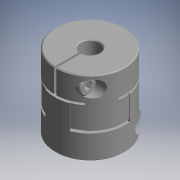
# Autodesk Inventor part: 562682 EAMC-30-32-8-14
Saved by Autodesk Inventor 2017.3 (Build 213256000, 256)
## iProperties
Part Number: 562682 EAMC-30-32-8-14
Material: Generic
Catalog Web Link: www.cadenas.de
Description: EAMC-Coupling
Vendor: FESTO
Document SubType Name: Modeling
Designer: partserver
Manufacturer: FESTO
Mass: 48 g
Surface Area: 90.1737 cm^2
Volume: 17.1118 cm^3
Density: 1 g/cm^3
Appearance: PSOLRGB-192-192-192
Category: PARTsolutions
Company: FESTO
Title: 562682 EAMC-30-32-8-14
Author: Cadenas PARTsolutions
Comments: Coupling
PSOL_IDENT_0: {$CADENAS_DATA\23d-libs\festo\parts\e\eamc\eamc.prj},183 {VTYP=3D},{NB=562682 EAMC-30-32-8-14},{LINA=
PSOL_IDENT_1: 562682 EAMC-30-32-8-14},{NN=EAMC},{DATE=08.03.2021 06:21:26},{GEOMDATE=08.03.2021 06:21:00},{VERSION=
PSOL_IDENT_2: },{LINEID=980},{WBVAR=},{WBNUMERIC=}  {NB=562682 EAMC-30-32-8-14},{LINA=562682 EAMC-30-32-8-14},{KT=
PSOL_IDENT_3: DUMMY},{TNR=562682},{TYP=EAMC-30-32-8-14},{INFO=},{CNSMASSEXACT=0.048},{VERS=7.000},{VERS2=0.000},{D=
PSOL_IDENT_4: 14},{D1=8.00},{D2=14.00},{D3=0.000},{D4=0.000},{L1=0.000},{L2=0.000},{L3=0.000},{L4=0.000},{L5=0.000
PSOL_IDENT_5: },{L6=0.000},{X=0.000},{EOLDATE=},{DI=14.200}
NB: 562682 EAMC-30-32-8-14
NN: EAMC
NT: Coupling
NBSYN: $TNR. $TYP.
LINA: 562682 EAMC-30-32-8-14
CATALOG: Festo
TNR: 562682
TYP: EAMC-30-32-8-14
CNSMASSEXACT: 0.048
D: 14
D1: 8
D2: 14
D3: 0
L1: 0
L2: 0
L3: 0
DI: 14.2
SUPPLIER: FESTO
ARTICLENO: 562682 EAMC-30-32-8-14
BOMINFO: 562682 EAMC-30-32-8-14
CREATOR: CADENAS GmbH
Autodesk Inventor part; units mm, degrees
sketch "Sketch_1" plane through (0, 0, 0) normal (1, 0, 0) x (0, 1, 0)
  line L0 (0, 10.3) -> (0, 0)
  line L1 (0, 0) -> (-15, 0)
  line L2 (-15, 0) -> (-15, 10.3)
  line L3 (-15, 10.3) -> (0, 10.3)
  line L4 (0, 10.3) -> (0, 0)
  constraints: 10 end point
revolve "Revolution1" add sketch "Sketch_1" angle 360 about axis through (0, 0, 10.3) along (0, 0, -1)
sketch "Sketch_2" plane through (0, 0, 9.3) normal (0, 0, 1) x (1, 0, 0)
  line L0 (-5.831, 14.8996) -> (-2.8531, 9.7417)
  arc A0 (-2.8531, 9.7417) -> (-0.9134, 8.7525) centre (-1.121, 10.7417) ccw
  arc A1 (0.9134, 8.7525) -> (-0.9134, 8.7525) centre (0, 0) ccw
  arc A2 (0.9134, 8.7525) -> (2.8531, 9.7417) centre (1.121, 10.7417) ccw
  line L1 (2.8531, 9.7417) -> (5.831, 14.8996)
  arc A3 (5.831, 14.8996) -> (-5.831, 14.8996) centre (0, 0) ccw
  constraints: 8 point on circle, 4 centre point, 4 end point
extrude "Extrusion1" add sketch "Sketch_2" along normal blind 11.4
sketch "Sketch_3" plane through (0, 0, 10.3) normal (0, 0, 1) x (1, 0, 0)
  arc A0 (-15.819, -2.4) -> (-9.9879, -12.4996) centre (0, 0) ccw
  line L0 (-9.9879, -12.4996) -> (-7.01, -7.3417)
  arc A1 (-7.01, -7.3417) -> (-7.1231, -5.1673) centre (-8.742, -6.3417) ccw
  arc A2 (-8.0366, -3.5852) -> (-7.1231, -5.1673) centre (0, 0) ccw
  arc A3 (-8.0366, -3.5852) -> (-9.8631, -2.4) centre (-9.8631, -4.4) ccw
  line L1 (-9.8631, -2.4) -> (-15.819, -2.4)
  constraints: 8 point on circle, 4 centre point, 4 end point
extrude "Extrusion2" add sketch "Sketch_3" along normal blind 10.4
sketch "Sketch_24" plane through (0, 0, 10.3) normal (0, 0, 1) x (1, 0, 0)
  arc A0 (7.1231, -5.1673) -> (7.01, -7.3417) centre (8.742, -6.3417) ccw
  line L0 (7.01, -7.3417) -> (9.9879, -12.4996)
  arc A1 (9.9879, -12.4996) -> (15.819, -2.4) centre (0, 0) ccw
  line L1 (15.819, -2.4) -> (9.8631, -2.4)
  arc A2 (9.8631, -2.4) -> (8.0366, -3.5852) centre (9.8631, -4.4) ccw
  arc A3 (7.1231, -5.1673) -> (8.0366, -3.5852) centre (0, 0) ccw
  constraints: 8 point on circle, 4 centre point, 4 end point
extrude "Extrusion3" add sketch "Sketch_24" along normal blind 10.4
sketch "Sketch_4" plane through (0, 0, 20.7) normal (0, 0, 1) x (1, 0, 0)
  arc A0 (-14.6202, 2.3) -> (-14.6202, -2.3) centre (0, 0) ccw
  line L0 (-14.6202, -2.3) -> (-10.016, -2.3)
  arc A1 (-8.1782, -3.511) -> (-10.016, -2.3) centre (-10.016, -4.3) ccw
  arc A2 (-8.1782, -3.511) -> (-7.1297, -5.327) centre (0, 0) ccw
  arc A3 (-6.9999, -7.5241) -> (-7.1297, -5.327) centre (-8.7319, -6.5241) ccw
  line L1 (-6.9999, -7.5241) -> (-9.302, -11.5115)
  arc A4 (-9.302, -11.5115) -> (-5.3182, -13.8115) centre (0, 0) ccw
  line L2 (-5.3182, -13.8115) -> (-3.0161, -9.8241)
  arc A5 (-1.0485, -8.838) -> (-3.0161, -9.8241) centre (-1.2841, -10.8241) ccw
  arc A6 (-1.0485, -8.838) -> (1.0485, -8.838) centre (0, 0) ccw
  arc A7 (3.0161, -9.8241) -> (1.0485, -8.838) centre (1.2841, -10.8241) ccw
  line L3 (3.0161, -9.8241) -> (5.3182, -13.8115)
  arc A8 (5.3182, -13.8115) -> (9.302, -11.5115) centre (0, 0) ccw
  line L4 (9.302, -11.5115) -> (6.9999, -7.5241)
  arc A9 (7.1297, -5.327) -> (6.9999, -7.5241) centre (8.7319, -6.5241) ccw
  arc A10 (7.1297, -5.327) -> (8.1782, -3.511) centre (0, 0) ccw
  arc A11 (10.016, -2.3) -> (8.1782, -3.511) centre (10.016, -4.3) ccw
  line L5 (10.016, -2.3) -> (14.6202, -2.3)
  arc A12 (14.6202, -2.3) -> (14.6202, 2.3) centre (0, 0) ccw
  line L6 (14.6202, 2.3) -> (10.016, 2.3)
  arc A13 (8.1782, 3.511) -> (10.016, 2.3) centre (10.016, 4.3) ccw
  arc A14 (8.1782, 3.511) -> (7.1297, 5.327) centre (0, 0) ccw
  arc A15 (6.9999, 7.5241) -> (7.1297, 5.327) centre (8.7319, 6.5241) ccw
  line L7 (6.9999, 7.5241) -> (9.302, 11.5115)
  arc A16 (9.302, 11.5115) -> (5.3182, 13.8115) centre (0, 0) ccw
  line L8 (5.3182, 13.8115) -> (3.0161, 9.8241)
  arc A17 (1.0485, 8.838) -> (3.0161, 9.8241) centre (1.2841, 10.8241) ccw
  arc A18 (1.0485, 8.838) -> (-1.0485, 8.838) centre (0, 0) ccw
  arc A19 (-3.0161, 9.8241) -> (-1.0485, 8.838) centre (-1.2841, 10.8241) ccw
  line L9 (-3.0161, 9.8241) -> (-5.3182, 13.8115)
  arc A20 (-5.3182, 13.8115) -> (-9.302, 11.5115) centre (0, 0) ccw
  line L10 (-9.302, 11.5115) -> (-6.9999, 7.5241)
  arc A21 (-7.1297, 5.327) -> (-6.9999, 7.5241) centre (-8.7319, 6.5241) ccw
  arc A22 (-7.1297, 5.327) -> (-8.1782, 3.511) centre (0, 0) ccw
  arc A23 (-10.016, 2.3) -> (-8.1782, 3.511) centre (-10.016, 4.3) ccw
  line L11 (-10.016, 2.3) -> (-14.6202, 2.3)
  constraints: 48 point on circle, 24 centre point, 24 end point
extrude "Extrusion4" add sketch "Sketch_4" against normal blind 9.4
sketch "Sketch_5" plane through (0, 0, 21.2) normal (0, 0, 1) x (1, 0, 0)
  circle A0 centre (6.132, -10.617) radius 1
  constraints: 1 centre point
extrude "Extrusion5" add sketch "Sketch_5" against normal blind 10.5
sketch "Sketch_6" plane through (0, 0, 21.2) normal (0, 0, 1) x (1, 0, 0)
  circle A0 centre (12.2606, 0.002) radius 1
  constraints: 1 centre point
extrude "Extrusion6" add sketch "Sketch_6" against normal blind 10.5
sketch "Sketch_25" plane through (0, 0, 21.2) normal (0, 0, 1) x (1, 0, 0)
  circle A0 centre (6.1286, 10.619) radius 1
  constraints: 1 centre point
extrude "Extrusion7" add sketch "Sketch_25" against normal blind 10.5
sketch "Sketch_26" plane through (0, 0, 21.2) normal (0, 0, 1) x (1, 0, 0)
  circle A0 centre (-6.132, 10.617) radius 1
  constraints: 1 centre point
extrude "Extrusion8" add sketch "Sketch_26" against normal blind 10.5
sketch "Sketch_27" plane through (0, 0, 21.2) normal (0, 0, 1) x (1, 0, 0)
  circle A0 centre (-12.2606, -0.002) radius 1
  constraints: 1 centre point
extrude "Extrusion9" add sketch "Sketch_27" against normal blind 10.5
sketch "Sketch_28" plane through (0, 0, 21.2) normal (0, 0, 1) x (1, 0, 0)
  circle A0 centre (-6.1286, -10.619) radius 1
  constraints: 1 centre point
extrude "Extrusion10" add sketch "Sketch_28" against normal blind 10.5
sketch "Sketch_7" plane through (0, 0, 11.3) normal (0, 0, 1) x (1, 0, 0)
  line L0 (-15.819, 2.4) -> (-9.8631, 2.4)
  arc A0 (-9.8631, 2.4) -> (-8.0366, 3.5852) centre (-9.8631, 4.4) ccw
  arc A1 (-7.1231, 5.1673) -> (-8.0366, 3.5852) centre (0, 0) ccw
  arc A2 (-7.1231, 5.1673) -> (-7.01, 7.3417) centre (-8.742, 6.3417) ccw
  line L1 (-7.01, 7.3417) -> (-9.9879, 12.4996)
  arc A3 (-9.9879, 12.4996) -> (-15.819, 2.4) centre (0, 0) ccw
  constraints: 8 point on circle, 4 centre point, 4 end point
extrude "Extrusion11" add sketch "Sketch_7" along normal blind 11
sketch "Sketch_8" plane through (0, 0, 11.3) normal (0, 0, 1) x (1, 0, 0)
  arc A0 (-5.831, -14.8996) -> (5.831, -14.8996) centre (0, 0) ccw
  line L0 (5.831, -14.8996) -> (2.8531, -9.7417)
  arc A1 (2.8531, -9.7417) -> (0.9134, -8.7525) centre (1.121, -10.7417) ccw
  arc A2 (-0.9134, -8.7525) -> (0.9134, -8.7525) centre (0, 0) ccw
  arc A3 (-0.9134, -8.7525) -> (-2.8531, -9.7417) centre (-1.121, -10.7417) ccw
  line L1 (-2.8531, -9.7417) -> (-5.831, -14.8996)
  constraints: 8 point on circle, 4 centre point, 4 end point
extrude "Extrusion12" add sketch "Sketch_8" along normal blind 11
sketch "Sketch_29" plane through (0, 0, 11.3) normal (0, 0, 1) x (1, 0, 0)
  arc A0 (7.01, 7.3417) -> (7.1231, 5.1673) centre (8.742, 6.3417) ccw
  arc A1 (8.0366, 3.5852) -> (7.1231, 5.1673) centre (0, 0) ccw
  arc A2 (8.0366, 3.5852) -> (9.8631, 2.4) centre (9.8631, 4.4) ccw
  line L0 (9.8631, 2.4) -> (15.819, 2.4)
  arc A3 (15.819, 2.4) -> (9.9879, 12.4996) centre (0, 0) ccw
  line L1 (9.9879, 12.4996) -> (7.01, 7.3417)
  constraints: 8 point on circle, 4 centre point, 4 end point
extrude "Extrusion13" add sketch "Sketch_29" along normal blind 11
sketch "Sketch_9" plane through (0, 0, 0) normal (1, 0, 0) x (0, 1, 0)
  line L0 (0, 32) -> (0, 21.7)
  line L1 (0, 21.7) -> (-15, 21.7)
  line L2 (-15, 21.7) -> (-15, 32)
  line L3 (-15, 32) -> (0, 32)
  line L4 (0, 32) -> (0, 21.7)
  constraints: 10 end point
revolve "Revolution2" add sketch "Sketch_9" angle 360 about axis through (0, 0, 32) along (0, 0, -1)
sketch "Sketch_10" plane through (0, 0, 0) normal (1, 0, 0) x (0, 1, 0)
  line L0 (0, 32) -> (0, 0)
  line L1 (-14.6, 32) -> (-17, 32)
  line L2 (-17, 32) -> (-17, 0)
  line L3 (-17, 0) -> (-14.6, 0)
  line L4 (-14.6, 0) -> (-15, 0.4)
  line L5 (-15, 0.4) -> (-15, 31.6)
  line L6 (-15, 31.6) -> (-14.6, 32)
  constraints: 14 end point
revolve "Revolution3" cut sketch "Sketch_10" angle 360 about axis through (0, 0, 32) along (0, 0, -1)
sketch "Sketch_11" plane through (0, 0, 0) normal (1, 0, 0) x (0, 1, 0)
  line L0 (0, 32) -> (0, 0)
  line L1 (0, 0) -> (-4.4, 0)
  line L2 (-4.4, 0) -> (-4, 0.4)
  line L3 (-4, 0.4) -> (-4, 9.8)
  line L4 (-4, 9.8) -> (-8.3, 9.8)
  arc A0 (-8.8, 10.3) -> (-8.3, 9.8) centre (-8.3, 10.3) ccw
  line L5 (-8.8, 10.3) -> (-8.8, 11.25)
  line L6 (-8.8, 11.25) -> (-7.1, 11.25)
  line L7 (-7.1, 11.25) -> (-7.1, 20.75)
  line L8 (-7.1, 20.75) -> (-8.8, 20.75)
  line L9 (-8.8, 20.75) -> (-8.8, 22.1)
  arc A1 (-8.3, 22.6) -> (-8.8, 22.1) centre (-8.3, 22.1) ccw
  line L10 (-8.3, 22.6) -> (-7, 22.6)
  line L11 (-7, 22.6) -> (-7, 31.6)
  line L12 (-7, 31.6) -> (-7.4, 32)
  line L13 (-7.4, 32) -> (0, 32)
  line L14 (0, 32) -> (0, 0)
  constraints: 30 end point, 4 point on circle, 2 centre point
revolve "Revolution4" cut sketch "Sketch_11" angle 360 about axis through (0, 0, 32) along (0, 0, -1)
sketch "Sketch_20" plane through (0, 0, 0) normal (0, 0, 1) x (1, 0, 0)
  line L0 (-0.5, -16) -> (0.5, -16)
  line L1 (0.5, -16) -> (0.5, 0)
  line L2 (0.5, 0) -> (-0.5, 0)
  line L3 (-0.5, 0) -> (-0.5, -16)
  constraints: 8 end point
extrude "Extrusion14" cut sketch "Sketch_20" along normal blind 10.3
sketch "Sketch_21" plane through (0, 0, 32) normal (0, 0, 1) x (1, 0, 0)
  line L0 (-0.5, 0) -> (0.5, 0)
  line L1 (0.5, 0) -> (0.5, 16)
  line L2 (0.5, 16) -> (-0.5, 16)
  line L3 (-0.5, 16) -> (-0.5, 0)
  constraints: 8 end point
extrude "Extrusion15" cut sketch "Sketch_21" against normal blind 10.3
sketch "Sketch_13" plane through (0, 0, 5.1) normal (0, 0, 1) x (1, 0, 0)
  line L0 (-16.5, -9.8) -> (13.5, -9.8)
  line L1 (13.5, -9.8) -> (13.5, -11.8)
  line L2 (13.5, -11.8) -> (13.121, -11.421)
  line L3 (13.121, -11.421) -> (-4.721, -11.421)
  line L4 (-4.721, -11.421) -> (-5.1, -11.8)
  line L5 (-5.1, -11.8) -> (-5.1, -13.3)
  line L6 (-5.1, -13.3) -> (-16.5, -13.3)
  line L7 (-16.5, -13.3) -> (-16.5, -9.8)
  line L8 (-16.5, -9.8) -> (13.5, -9.8)
  constraints: 18 end point
revolve "Revolution5" cut sketch "Sketch_13" angle 360 about axis through (-16.5, -9.8, 5.1) along (-1, 0, 0)
thread "Thread1" size "M4x0.7" class "6H" standard "ISO Metric profile" length 17.842
sketch "Sketch_15" plane through (0, 0, 5.1) normal (0, 0, 1) x (1, 0, 0)
  line L0 (-9.1, -9.8) -> (6.9, -9.8)
  line L1 (6.9, -9.8) -> (6.9, -11.8)
  line L2 (6.9, -11.8) -> (-5.1, -11.8)
  line L3 (-5.1, -11.8) -> (-5.1, -13.3)
  line L4 (-5.1, -13.3) -> (-8.7, -13.3)
  line L5 (-8.7, -13.3) -> (-9.1, -12.9)
  line L6 (-9.1, -12.9) -> (-9.1, -9.8)
  line L7 (-9.1, -9.8) -> (6.9, -9.8)
  constraints: 16 end point
revolve "Revolution6" add sketch "Sketch_15" angle 360 about axis through (-9.1, -9.8, 5.1) along (-1, 0, 0)
sketch "Sketch_14" plane through (0, 0, 26.9) normal (0, 0, 1) x (1, 0, 0)
  line L0 (-16.5, 9.8) -> (13.5, 9.8)
  line L1 (13.5, 9.8) -> (13.5, 7.8)
  line L2 (13.5, 7.8) -> (13.121, 8.179)
  line L3 (13.121, 8.179) -> (-4.721, 8.179)
  line L4 (-4.721, 8.179) -> (-5.1, 7.8)
  line L5 (-5.1, 7.8) -> (-5.1, 5.8)
  line L6 (-5.1, 5.8) -> (-16.5, 5.8)
  line L7 (-16.5, 5.8) -> (-16.5, 9.8)
  line L8 (-16.5, 9.8) -> (13.5, 9.8)
  constraints: 18 end point
revolve "Revolution7" cut sketch "Sketch_14" angle 360 about axis through (-16.5, 9.8, 26.9) along (-1, 0, 0)
thread "Thread2" size "M4x0.7" class "6H" standard "ISO Metric profile" length 17.842
sketch "Sketch_16" plane through (0, 0, 26.9) normal (0, 0, 1) x (1, 0, 0)
  line L0 (-9.1, 9.8) -> (6.9, 9.8)
  line L1 (6.9, 9.8) -> (6.9, 7.8)
  line L2 (6.9, 7.8) -> (-5.1, 7.8)
  line L3 (-5.1, 7.8) -> (-5.1, 6.3)
  line L4 (-5.1, 6.3) -> (-8.7, 6.3)
  line L5 (-8.7, 6.3) -> (-9.1, 6.7)
  line L6 (-9.1, 6.7) -> (-9.1, 9.8)
  line L7 (-9.1, 9.8) -> (6.9, 9.8)
  constraints: 16 end point
revolve "Revolution8" add sketch "Sketch_16" angle 360 about axis through (-9.1, 9.8, 26.9) along (-1, 0, 0)
sketch "Sketch_17" plane through (-9.1, 0, 0) normal (1, 0, 0) x (0, 0, -1)
  line L0 (-6.6, -8.934) -> (-6.6, -10.666)
  line L1 (-6.6, -10.666) -> (-5.1, -11.5321)
  line L2 (-5.1, -11.5321) -> (-3.6, -10.666)
  line L3 (-3.6, -10.666) -> (-3.6, -8.934)
  line L4 (-3.6, -8.934) -> (-5.1, -8.0679)
  line L5 (-5.1, -8.0679) -> (-6.6, -8.934)
  constraints: 12 end point
extrude "Extrusion16" cut sketch "Sketch_17" along normal blind 2
sketch "Sketch_18" plane through (-9.1, 0, 0) normal (1, 0, 0) x (0, 0, -1)
  line L0 (-28.4, 10.666) -> (-28.4, 8.934)
  line L1 (-28.4, 8.934) -> (-26.9, 8.0679)
  line L2 (-26.9, 8.0679) -> (-25.4, 8.934)
  line L3 (-25.4, 8.934) -> (-25.4, 10.666)
  line L4 (-25.4, 10.666) -> (-26.9, 11.5321)
  line L5 (-26.9, 11.5321) -> (-28.4, 10.666)
  constraints: 12 end point
extrude "Extrusion17" cut sketch "Sketch_18" along normal blind 2
ref_plane "KUP_XY" through (0, 0, 0) normal (0, 0, 1) x (1, 0, 0)
ref_plane "KUP_YZ" through (0, 0, 0) normal (1, 0, 0) x (0, 1, 0)
ref_plane "KUP_ZX" through (0, 0, 0) normal (0, 1, 0) x (0, 0, 1)
ref_plane "LINKS_XY" through (0, 0, 32) normal (0, 0, 1) x (1, 0, 0)
ref_plane "LINKS_YZ" through (0, 0, 32) normal (1, 0, 0) x (0, 1, 0)
ref_plane "LINKS_ZX" through (0, 0, 32) normal (0, 1, 0) x (0, 0, 1)
ref_plane "RECHTS_XY" through (0, 0, 0) normal (0, 0, 1) x (1, 0, 0)
ref_plane "RECHTS_YZ" through (0, 0, 0) normal (1, 0, 0) x (0, 1, 0)
ref_plane "RECHTS_ZX" through (0, 0, 0) normal (0, 1, 0) x (0, 0, 1)
body "Solid1"
